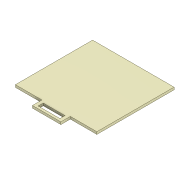
# Autodesk Inventor part: pokrywa
Saved by Autodesk Inventor 2021 (Build 250183000, 183)
## iProperties
Created: 2022-09-09
Part Number: pokrywa
Material: Generic
Document SubType Name: Modeling
Designer: agnpi
Density: 1 g/cm^3
Appearance: Smooth - Ash
Author: agnpi
Autodesk Inventor part; units mm, degrees
ref_plane "YZ Plane" through (0, 0, 0) normal (1, 0, 0) x (0, 1, 0)
ref_plane "XZ Plane" through (0, 0, 0) normal (0, 1, 0) x (-1, 0, 0)
ref_plane "XY Plane" through (0, 0, 0) normal (0, 0, 1) x (1, 0, 0)
sketch "Sketch1" plane through (0, 0, 0) normal (0, 1, 0) x (-1, 0, 0)
  line L0 (120.4, 0) -> (-120.4, 0) projected
  line L1 (0, -117.6) -> (0, 117.6) projected
  line L2 (-86, 84) -> (86, 84)
  line L3 (86, 84) -> (86, -84)
  line L4 (86, -84) -> (-86, -84)
  line L5 (-86, -84) -> (-86, 84)
  line L6 (-86, 84) -> (86, -84) construction
  line L7 (86, 84) -> (-86, -84) construction
  point P0 (0, 0)
  dimension "d0" = 172
  dimension "d1" = 168
  constraints: 12 end point, 2 midpoint, 2 parallel, 1 horizontal, 1 perpendicular
  measures "d0" distance of L3.end L4.end
  measures "d1" distance of L2.end L3.end
extrude "Extrusion1" add sketch "Sketch1" along normal blind 9
sketch "Sketch2" plane through (-86, 0, 84) normal (0, 0, 1) x (1, 0, 0)
  line L0 (172, 9) -> (0, 9) projected
  line L1 (172, 0) -> (0, 0) projected
  line L2 (56, 9) -> (116, 9)
  line L3 (116, 9) -> (116, 0)
  line L4 (116, 0) -> (56, 0)
  line L5 (56, 0) -> (56, 9)
  point P0 (86, 0)
  dimension "d4" = 60
  dimension "d5" = 30
  constraints: 8 end point, 2 parallel, 2 point on line, 1 horizontal, 1 perpendicular
  measures "d4" distance between parallel lines of L3 L5
  measures "d5" distance from line of point (86, 0) L3
extrude "Extrusion2" add sketch "Sketch2" along normal blind 20
sketch "Sketch3" plane through (0, 9, 0) normal (0, 1, 0) x (1, 0, 0)
  line L0 (-23, -88.1983) -> (23, -88.1983)
  line L1 (23, -88.1983) -> (23, -99)
  line L2 (23, -99) -> (-23, -99)
  line L3 (-23, -99) -> (-23, -88.1983)
  line L4 (30, -84) -> (30, -104) projected
  line L5 (30, -104) -> (-30, -104) projected
  line L6 (-30, -84) -> (-30, -104) projected
  line L7 (30, -84) -> (86, -84) projected
  point P0 (0, 0)
  dimension "d8" = 7
  dimension "d9" = 5
  dimension "d10" = 7
  dimension "d11" = 4.1983
  constraints: 8 end point, 2 parallel, 1 horizontal, 1 perpendicular
  measures "d8" distance between parallel lines of L4 L1
  measures "d9" distance between parallel lines of L5 L2
  measures "d10" distance between parallel lines of L6 L3
  measures "d11" distance between parallel lines of L7 L0
extrude "Extrusion3" cut sketch "Sketch3" against normal blind 20
move faces "Move1" translate (0, -4, 0) faces at (-10, 9, -28)
move faces "Move2" translate (0, 0, 5) faces at (28.6667, 1.6667, -84)
body "Solid1"
